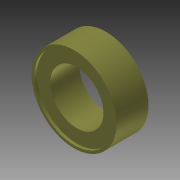
# Autodesk Inventor part: Dewalt Drill Shaft Bearing 1in x ..625 x 375
Saved by Autodesk Inventor 2012 (Build 160160000, 160)
## iProperties
Created: 2012-07-04
Part Number: Dewalt Drill Shaft Bearing 1in x ..625 x 375
Material: Default
Document SubType Name: Modeling
Designer: Bruce
Density: 1 g/cm^3
Author: Bruce
Autodesk Inventor part; units mm, degrees
ref_plane "YZ Plane" through (0, 0, 0) normal (1, 0, 0) x (0, 1, 0)
ref_plane "XZ Plane" through (0, 0, 0) normal (0, 1, 0) x (-1, 0, 0)
ref_plane "XY Plane" through (0, 0, 0) normal (0, 0, 1) x (1, 0, 0)
sketch "Sketch1" plane through (0, 0, 0) normal (0, 0, 1) x (1, 0, 0)
  circle A0 centre (0, 0) radius 12.7
  circle A1 centre (0, 0) radius 7.9375
  circle A2 centre (0, 0) radius 11.9062
  dimension "d0" = 25.4
  dimension "d1" = 23.8125
  dimension "d3" = 15.875
  constraints: 3 centre point, 3 coincident
  measures "d0" diameter of A0
  measures "d1" diameter of A2
  measures "d3" diameter of A1
extrude "Extrusion1" add sketch "Sketch1" against normal blind 9.525 contours A0 | A2
extrude "Extrusion2" cut sketch "Sketch1" against normal blind 0.8255 contours A2
body "Solid1"
